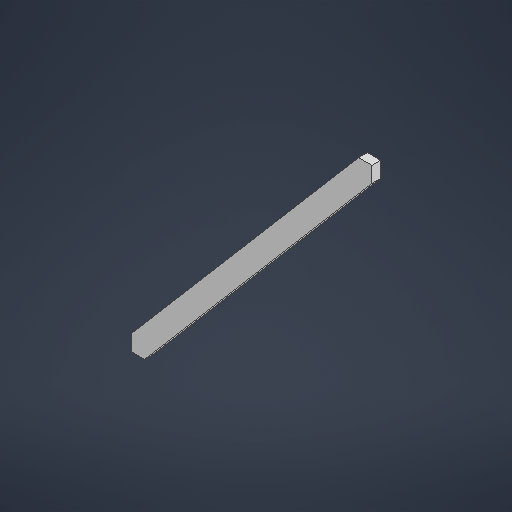
# Autodesk Inventor part: S_2x4x63.127
Saved by Autodesk Inventor 2026 (Build 300175000, 175)
## iProperties
Created: 2025-09-02
Part Number: S_2x4x63.127
Material: Generic
Document SubType Name: Modeling
Designer: trott
Density: 1 g/cm^3
Appearance: Default
Author: trott
Autodesk Inventor part; units mm, degrees
ref_plane "YZ Plane" through (0, 0, 0) normal (1, 0, 0) x (0, 1, 0)
ref_plane "XZ Plane" through (0, 0, 0) normal (0, 1, 0) x (-1, 0, 0)
ref_plane "XY Plane" through (0, 0, 0) normal (0, 0, 1) x (1, 0, 0)
sketch "Sketch1" plane through (0, 0, 0) normal (0, 0, 1) x (1, 0, 0)
  line L0 (-520.7, -609.6) -> (520.7, -609.6)
  line L1 (520.7, -609.6) -> (520.7, 609.6)
  line L2 (520.7, 609.6) -> (-520.7, 609.6)
  line L3 (-520.7, 609.6) -> (-520.7, -609.6)
  line L4 (-520.7, -609.6) -> (520.7, 609.6) construction
  line L5 (520.7, -609.6) -> (-520.7, 609.6) construction
  line L6 (28.8696, -33.7986) -> (-28.8696, 33.7986)
  line L7 (-520.7, -542.0028) -> (462.9607, 609.6)
  line L8 (-462.9607, -609.6) -> (520.7, 542.0028)
  point P0 (0, 0)
  dimension "d0" = 1219.2
  dimension "d1" = 1041.4
  dimension "d3" = 88.9
  constraints: 18 end point, 5 midpoint, 4 parallel, 3 point on line, 1 horizontal, 1 perpendicular
  measures "d0" distance of L0.end L1.end
  measures "d1" distance of L1.end L2.end
  measures "d3" distance of L6.start L6.end
extrude "Extrusion1" add sketch "Sketch1" along normal blind 38.1 contours L3 L7 L6 L8 L0 | L6 L7 L2 L1 L8
body "Solid1"
